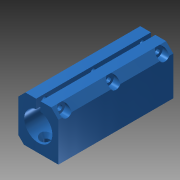
# Autodesk Inventor part: ZAxisCarriageLeft
Saved by Autodesk Inventor 2015 SP1 (Build 190203100, 203)
## iProperties
Category: Print
Created: 2014-12-10
Part Number: ZAxisCarriageLeft
Material: Generic
Document SubType Name: Modeling
Designer: Jack
Density: 1 g/cm^3
Appearance: Cyan
Mass: 42.0238 g
Surface Area: 164.818 cm^2
Volume: 42.0238 cm^3
Catalog Web Link: N/A
Author: Jack
Title: Z Axis Carraige Left
Autodesk Inventor part; units mm, degrees
ref_plane "YZ Plane" through (0, 0, 0) normal (1, 0, 0) x (0, 1, 0)
ref_plane "XZ Plane" through (0, 0, 0) normal (0, 1, 0) x (-1, 0, 0)
ref_plane "XY Plane" through (0, 0, 0) normal (0, 0, 1) x (1, 0, 0)
sketch "Sketch1" plane through (0, 0, 0) normal (0, 1, 0) x (-1, 0, 0)
  arc A0 (-1.5, 9.6845) -> (1.5, 9.6845) centre (0, 0) ccw
  line L0 (14, -16) -> (14, 11)
  line L1 (14, 11) -> (9, 16)
  line L2 (9, 16) -> (1.5, 16)
  line L3 (1.5, 16) -> (1.5, 9.6845)
  line L4 (-1.5, 9.6845) -> (-1.5, 16)
  line L5 (-1.5, 16) -> (-9, 16)
  line L6 (-9, 16) -> (-14, 11)
  line L7 (-14, 11) -> (-14, -16)
  line L8 (14, -16) -> (-14, -16)
  dimension "d0" = 19.6
  dimension "d1" = 135
  dimension "d2" = 135
  dimension "d3" = 14
  dimension "d4" = 14
  dimension "d5" = 16
  dimension "d6" = 16
  dimension "d7" = 1.5
  dimension "d8" = 5
  constraints: 18 end point, 2 equal length, 2 parallel, 2 perpendicular, 2 point on circle, 2 point on line, 1 centre point, 1 coincident, 1 horizontal, 1 vertical
  measures "d0" diameter of A0
  measures "d1" angle of L0 L1
  measures "d2" angle of L7 L6
  measures "d3" distance from line of point (0, 0) L0
  measures "d4" distance from line of point (0, 0) L7
  measures "d5" distance from line of point (0, 0) L5
  measures "d6" distance from line of point (0, 0) L8
  measures "d7" distance from line of point (0, 0) L3
  measures "d8" horizontal distance of L6.end L5.end
extrude "Extrusion1" add sketch "Sketch1" along normal blind 80
sketch "Sketch4" plane through (14, 0, 11) normal (1, 0, 0) x (0, 0, -1)
  line L0 (0, 0) -> (0, 80) projected
  line L1 (-5, 0) -> (0, 0) projected
  line L2 (0, 0) -> (0, 80) projected
  line L3 (-5, 80) -> (0, 80) projected
  line L4 (-5, 0) -> (-5, 80) projected
  circle A0 centre (-1.7, 74) radius 1.75
  circle A1 centre (-1.7, 40) radius 1.75
  circle A2 centre (-1.7, 6) radius 1.75
  point P0 (11, 0)
  dimension "d20" = 3.5
  dimension "d21" = 6
  dimension "d22" = 6
  dimension "d23" = 40
  dimension "d24" = 1.7
  constraints: 3 centre point, 2 equal radius, 2 vertical alignment
  measures "d20" diameter of A2
  measures "d21" distance from line of L3 A0.centre
  measures "d22" distance from line of L1 A2.centre
  measures "d23" distance from line of L1 A1.centre
  measures "d24" distance from line of L0 A0.centre
extrude "Extrusion4" cut sketch "Sketch4" against normal blind 26 contours A2 L0 | L0 A2 | A1 L0 | L0 A1 | A0 L0 | L0 A0
sketch "Sketch5" plane through (14, 0, 11) normal (1, 0, 0) x (0, 0, -1)
  arc A0 (0, 74.4153) -> (0, 73.5847) centre (-1.7, 74) ccw projected
  circle A1 centre (-1.7, 74) radius 1.75 projected
  arc A2 (0, 40.4153) -> (0, 39.5847) centre (-1.7, 40) ccw projected
  circle A3 centre (-1.7, 40) radius 1.75 projected
  arc A4 (0, 6.4153) -> (0, 5.5847) centre (-1.7, 6) ccw projected
  circle A5 centre (-1.7, 6) radius 1.75 projected
  circle A6 centre (-1.7, 74) radius 3.65
  circle A7 centre (-1.7, 40) radius 3.65
  circle A8 centre (-1.7, 6) radius 3.65
  arc A9 (0, 5.5847) -> (0, 6.4153) centre (-1.7, 6) ccw projected
  arc A10 (0, 39.5847) -> (0, 40.4153) centre (-1.7, 40) ccw projected
  arc A11 (0, 73.5847) -> (0, 74.4153) centre (-1.7, 74) ccw projected
  point P0 (11, 0)
  dimension "d27" = 7.3
  dimension "d28" = 7.3
  dimension "d29" = 7.3
  constraints: 3 centre point, 3 coincident
  measures "d27" diameter of A6
  measures "d28" diameter of A7
  measures "d29" diameter of A8
extrude "Extrusion5" cut sketch "Sketch5" against normal blind 5
sketch "Sketch6" plane through (-14, 0, 11) normal (-1, 0, 0) x (0, 0, 1)
  circle A0 centre (1.7, 74) radius 1.75 projected
  circle A1 centre (1.7, 40) radius 1.75 projected
  circle A2 centre (1.7, 6) radius 1.75 projected
  line L0 (4.45, 75.5877) -> (4.45, 72.4123)
  line L1 (4.45, 72.4123) -> (1.7, 70.8246)
  line L2 (1.7, 70.8246) -> (-1.05, 72.4123)
  line L3 (-1.05, 72.4123) -> (-1.05, 75.5877)
  line L4 (-1.05, 75.5877) -> (1.7, 77.1754)
  line L5 (1.7, 77.1754) -> (4.45, 75.5877)
  line L6 (4.45, 41.5877) -> (4.45, 38.4123)
  line L7 (4.45, 38.4123) -> (1.7, 36.8246)
  line L8 (1.7, 36.8246) -> (-1.05, 38.4123)
  line L9 (-1.05, 38.4123) -> (-1.05, 41.5877)
  line L10 (-1.05, 41.5877) -> (1.7, 43.1754)
  line L11 (1.7, 43.1754) -> (4.45, 41.5877)
  line L12 (4.45, 7.5877) -> (4.45, 4.4123)
  line L13 (4.45, 4.4123) -> (1.7, 2.8246)
  line L14 (1.7, 2.8246) -> (-1.05, 4.4123)
  line L15 (-1.05, 4.4123) -> (-1.05, 7.5877)
  line L16 (-1.05, 7.5877) -> (1.7, 9.1754)
  line L17 (1.7, 9.1754) -> (4.45, 7.5877)
  point P0 (-11, 0)
  point P1 (1.7, 74)
  point P2 (1.7, 40)
  point P3 (1.7, 6)
  dimension "d32" = 5.5
  constraints: 36 end point, 3 coincident, 3 vertical, 2 collinear, 39 other
  measures "d32" distance between parallel lines of L15 L12
extrude "Extrusion6" cut sketch "Sketch6" against normal blind 5 contours A0 | A1 | A2 | L0 L1 L2 L3 L4 L5 | L6 L7 L8 L9 L10 L11 | L12 L13 L14 L15 L16 L17
chamfer "Chamfer2" distance 4 angle 45 1 edges at (-14, 40, -16)
sketch "Sketch9" plane through (14, 0, -16) normal (0, 0, -1) x (-1, 0, 0)
  line L0 (0, 80) -> (24, 80) projected
  line L1 (0, 0) -> (24, 0) projected
  line L2 (28, 0) -> (28, 80) projected
  circle A0 centre (14, 74) radius 2.25
  circle A1 centre (14, 40) radius 2.25
  circle A2 centre (14, 6) radius 2.25
  point P0 (14, 0)
  dimension "d51" = 4.5
  dimension "d52" = 14
  dimension "d53" = 6
  dimension "d54" = 6
  dimension "d55" = 40
  constraints: 3 centre point, 2 equal radius, 2 vertical alignment
  measures "d51" diameter of A0
  measures "d52" distance from line of L2 A2.centre
  measures "d53" distance from line of A2.centre L1
  measures "d54" distance from line of L0 A0.centre
  measures "d55" distance from line of L1 A1.centre
extrude "Extrusion9" cut sketch "Sketch9" against normal up to next
chamfer "Chamfer3" distance 2.2 angle 45 3 edges at (2.25, 73.9963, -9.5382) (2.25, 39.9963, -9.5382) (2.25, 5.9963, -9.5382)
sketch "Sketch10" plane through (0, 80, 0) normal (0, 1, 0) x (1, 0, 0)
  line L0 (-14, 12) -> (-10, 16) projected
  line L1 (-14, 12) -> (-14, -11) projected
  line L2 (-14, -11) -> (-9, -16) projected
  line L3 (-9, -16) -> (-1.5, -16) projected
  line L4 (-1.5, -16) -> (-1.5, -9.6845) projected
  arc A0 (1.5, -9.6845) -> (-1.5, -9.6845) centre (0, 0) ccw projected
  line L5 (1.5, -9.6845) -> (1.5, -16) projected
  line L6 (1.5, -16) -> (9, -16) projected
  line L7 (9, -16) -> (14, -11) projected
  line L8 (14, -11) -> (14, 16) projected
  line L9 (14, 16) -> (-10, 16) projected
  line L10 (-14, -1) -> (-22, -1)
  line L11 (-22, -1) -> (-22, 1)
  line L12 (-22, 1) -> (-14, 1)
  line L13 (-14, 12) -> (-14, -11) projected
  dimension "d61" = 1
  dimension "d62" = 1
  dimension "d63" = 8
  constraints: 6 end point, 2 perpendicular, 2 point on line, 1 horizontal
  measures "d61" distance from line of A0.centre L10
  measures "d62" distance from line of A0.centre L12
  measures "d63" distance between parallel lines of L1 L11
extrude "Extrusion10" add sketch "Sketch10" against normal blind 10 contours L1 L10 L11 L12
chamfer "Chamfer4" distance 5 angle 45 1 edges at (-22, 70, 0)
body "Solid1"
